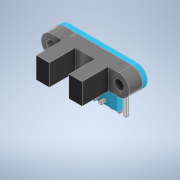
# Autodesk Inventor part: Оптический датчик
Saved by Autodesk Inventor 2023 (Build 270158000, 158)
## iProperties
Created: 2022-11-10
Part Number: Оптический датчик
Material: Типовые
Document SubType Name: Modeling
Designer: Admin
Density: 1 g/cm^3
Appearance: Резина — черная
Author: Admin
Autodesk Inventor part; units mm, degrees
ref_plane "YZ Plane" through (0, 0, 0) normal (1, 0, 0) x (0, 1, 0)
ref_plane "XZ Plane" through (0, 0, 0) normal (0, 1, 0) x (-1, 0, 0)
ref_plane "XY Plane" through (0, 0, 0) normal (0, 0, 1) x (1, 0, 0)
sketch "Эскиз1" plane through (0, 0, 0) normal (0, 0, 1) x (1, 0, 0)
  circle A0 centre (0, 0) radius 1.5
  circle A1 centre (20.6, 0) radius 1.5
  line L0 (0.05, 0) -> (20.55, 0) construction
  line L1 (0.05, -3.25) -> (20.55, -3.25)
  line L2 (20.55, 3.25) -> (0.05, 3.25)
  arc A2 (0.05, 3.25) -> (0.05, -3.25) centre (0.05, 0) ccw
  arc A3 (20.55, -3.25) -> (20.55, 3.25) centre (20.55, 0) ccw
  line L3 (10.3, 0) -> (10.3, 1.5) construction
  line L4 (4.3, -3.25) -> (16.3, -3.25)
  line L5 (16.3, -3.25) -> (16.3, -11.35)
  line L6 (16.3, -11.35) -> (4.3, -11.35)
  line L7 (4.3, -11.35) -> (4.3, -3.25)
  point P0 (1.5, 0)
  point P1 (-1.5, 0)
  point P2 (19.1, 0)
  point P3 (22.1, 0)
  point P4 (-3.2, 0)
  point P5 (23.8, 0)
  point P6 (10.3, -11.35)
  dimension "d2" = 3
  dimension "d3" = 20.6
  dimension "d4" = 17.6
  dimension "d5" = 23.6
  dimension "d6" = 6.5
  dimension "d7" = 27
  dimension "d8" = 14.6
  dimension "d9" = 12
  constraints: 18 end point, 10 point on circle, 7 horizontal alignment, 4 centre point, 4 tangent, 3 parallel, 2 horizontal, 2 midpoint, 1 coincident, 1 equal radius, 1 perpendicular, 1 point on line, 1 vertical, 1 vertical alignment, 1 other
  measures "d2" diameter of A1
  measures "d3" distance of point (0, 0) A1.centre
  measures "d4" distance of A0.start A1.start
  measures "d5" distance of A1.end A0.end
  measures "d6" distance between parallel lines of L1 L2
  measures "d7" distance of point (-3.2, 0) point (23.8, 0)
  measures "d8" distance between parallel lines of L2 L6
  measures "d9" distance between parallel lines of L7 L5
extrude "Выдавливание1" add sketch "Эскиз1" against normal blind 1.5
extrude "Выдавливание2" add sketch "Эскиз1" along normal blind 4 separate body contours A2 L2 A3 L1
sketch "Эскиз2" plane through (0, 0, 4) normal (0, 0, 1) x (1, 0, 0)
  line L0 (3.3, 3.25) -> (7.3, 3.25)
  line L1 (7.3, 3.25) -> (7.3, -3.25)
  line L2 (7.3, -3.25) -> (3.3, -3.25)
  line L3 (3.3, -3.25) -> (3.3, 3.25)
  line L4 (20.55, -3.25) -> (16.3, -3.25) projected
  line L5 (13.3, 3.25) -> (17.3, 3.25)
  line L6 (17.3, 3.25) -> (17.3, -3.25)
  line L7 (17.3, -3.25) -> (13.3, -3.25)
  line L8 (13.3, -3.25) -> (13.3, 3.25)
  line L9 (20.55, 3.25) -> (0.05, 3.25) projected
  line L10 (0.05, -3.25) -> (20.55, -3.25) projected
  line L11 (0.05, 3.25) -> (20.55, 3.25) projected
  line L12 (10.3, 3.25) -> (10.3, 1.8468) construction
  point P0 (0, 0)
  dimension "d14" = 14
  dimension "d15" = 6
  constraints: 18 end point, 5 point on line, 4 parallel, 2 horizontal, 2 perpendicular, 1 collinear, 1 midpoint, 1 vertical, 1 other
  measures "d14" distance between parallel lines of L3 L6
  measures "d15" distance between parallel lines of L8 L1
extrude "Выдавливание3" add sketch "Эскиз2" along normal blind 8 contours L0 L1 L2 L3 | L5 L6 L4 L7 L8 bodies 2
sketch "Эскиз3" plane through (0, 0, -1.5) normal (0, 0, -1) x (-1, 0, 0)
  line L0 (-16.3, -11.35) -> (-4.3, -11.35) projected
  line L1 (-13.8, -11.35) -> (-6.8, -11.35)
  line L2 (-6.8, -11.35) -> (-6.8, -8.85)
  line L3 (-6.8, -8.85) -> (-13.8, -8.85)
  line L4 (-13.8, -8.85) -> (-13.8, -11.35)
  point P0 (0, 0)
  point P1 (-10.3, -11.35)
  point P2 (-10.3, -11.35)
  point P3 (-10.3, -11.35)
  dimension "d18" = 2.5
  dimension "d19" = 7
  constraints: 8 end point, 3 midpoint, 2 coincident, 2 parallel, 1 horizontal, 1 perpendicular, 1 point on line
  measures "d18" distance between parallel lines of L0 L3
  measures "d19" distance of L2.end L3.end
extrude "Выдавливание4" add sketch "Эскиз3" along normal blind 2.5 separate body
ref_plane "РабПлоскость1" through (12.3, -11.35, -1.5) normal (1, 0, 0) x (0, 0, -1)
sketch "Эскиз4" plane through (12.3, -11.35, -1.5) normal (1, 0, 0) x (0, 0, -1)
  line L0 (-3, 1.25) -> (4.5, 1.25)
  line L1 (5, 0.75) -> (5, -6.25)
  line L2 (-1.5, 0) -> (-1.5, 8.1) projected
  line L3 (2.5, 2.5) -> (2.5, 0) projected
  arc A0 (5, 0.75) -> (4.5, 1.25) centre (4.5, 0.75) ccw
  point P0 (-1.5, 11.35)
  point P1 (5, 1.25)
  point P2 (2.5, 1.25)
  dimension "d23" = 8
  dimension "d24" = 1.5
  dimension "d26" = 0.5
  dimension "d37" = 7
  constraints: 4 end point, 3 point on line, 2 point on circle, 2 tangent, 1 centre point, 1 horizontal, 1 midpoint, 1 perpendicular
  measures "d23" distance of L0.start point (5, 1.25)
  measures "d24" distance from line of L2 L0.start
  measures "d26" radius of A0
  measures "d37" distance of L1.start L1.end
ref_plane "РабПлоскость2" through (12.3, -10.1, 1.5) normal (0, 0, 1) x (1, 0, 0)
sketch "Эскиз5" plane through (12.3, -10.1, 1.5) normal (0, 0, 1) x (1, 0, 0)
  line L0 (-0.375, 0.375) -> (0.375, 0.375)
  line L1 (0.375, 0.375) -> (0.375, -0.375)
  line L2 (0.375, -0.375) -> (-0.375, -0.375)
  line L3 (-0.375, -0.375) -> (-0.375, 0.375)
  line L4 (-0.375, 0.375) -> (0.375, -0.375) construction
  line L5 (0.375, 0.375) -> (-0.375, -0.375) construction
  point P0 (-12.3, 10.1)
  point P1 (0, 0)
  point P2 (0, 0)
  point P3 (0, 0)
  point P4 (0, 0)
  point P5 (0, 0)
  dimension "d25" = 0.75
  constraints: 12 end point, 3 midpoint, 2 parallel, 2 perpendicular, 1 coincident, 1 horizontal
  measures "d25" distance of L0.end L1.end
sweep "Сдвиг1" cut profiles "Эскиз5" path "Эскиз4" bodies 1 3 path curves L0 A0 L1
pattern_linear "Прямоуг.массив1" count 3 spacing 2 along (-1, 0, 0) of "Сдвиг1" bodies 3 1
sweep "Сдвиг2" add profiles "Эскиз5" path "Эскиз4" separate body path curves L0 A0 L1
pattern_linear "Прямоуг.массив2" count 3 spacing 2 along (-1, 0, 0) of "Сдвиг2" bodies 4
